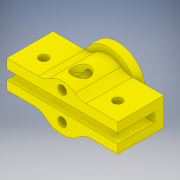
# Autodesk Inventor part: middledownthrustmt
Saved by Autodesk Inventor 2017 (Build 210142000, 142)
## iProperties
Created: 2017-08-12
Part Number: middledownthrustmt
Material: Generic
Document SubType Name: Modeling
Designer: Kai
Density: 1 g/cm^3
Appearance: Default
Author: Kai
Autodesk Inventor part; units mm, degrees
ref_plane "YZ Plane" through (0, 0, 0) normal (1, 0, 0) x (0, 1, 0)
ref_plane "XZ Plane" through (0, 0, 0) normal (0, 1, 0) x (-1, 0, 0)
ref_plane "XY Plane" through (0, 0, 0) normal (0, 0, 1) x (1, 0, 0)
sketch "Sketch1" plane through (0, 0, 0) normal (0, 0, 1) x (1, 0, 0)
  circle A0 centre (0, 0) radius 19.05
  dimension "d5" = 38.1
  constraints: 1 centre point
  measures "d5" diameter of A0
extrude "Extrusion1" add sketch "Sketch1" along normal blind 6.35
sketch "Sketch2" plane through (0, 0, 6.35) normal (0, 0, 1) x (1, 0, 0)
  line L0 (38.1, 9.525) -> (38.1, -9.525)
  line L1 (-38.1, -9.525) -> (-38.1, 9.525)
  line L2 (-34.9943, 0) -> (35.154, 0) construction
  line L3 (-38.1, 9.525) -> (-16.324, 9.525)
  line L4 (16.324, 9.525) -> (38.1, 9.525)
  line L5 (38.1, -9.525) -> (19.8184, -9.525)
  line L6 (-19.8184, -9.525) -> (-38.1, -9.525)
  arc A0 (-11.366, -12.7462) -> (11.366, -12.7462) centre (0, 0) ccw
  arc A1 (8.806, 11.9893) -> (-8.806, 11.9893) centre (0, 0) ccw
  arc A2 (-16.324, 9.525) -> (-8.806, 11.9893) centre (-16.324, 22.225) ccw
  arc A3 (8.806, 11.9893) -> (16.324, 9.525) centre (16.324, 22.225) ccw
  arc A4 (19.8184, -9.525) -> (11.366, -12.7462) centre (19.8184, -22.225) ccw
  arc A5 (-11.366, -12.7462) -> (-19.8184, -9.525) centre (-19.8184, -22.225) ccw
  point P0 (-11.4265, 9.525)
  point P1 (14.1749, -9.525)
  point P2 (-14.1749, -9.525)
  point P3 (11.4265, 9.525)
  dimension "d8" = 76.2
  dimension "d9" = 19.05
  dimension "d10" = 38.1
  dimension "d11" = 12.7
  dimension "d18" = 19.05
  constraints: 16 point on circle, 14 end point, 8 tangent, 6 centre point, 5 parallel, 4 point on line, 3 equal radius, 3 horizontal, 2 perpendicular, 1 coincident, 1 other
  measures "d8" distance of L0.end L1.start
  measures "d9" distance of L0.start L0.end
  measures "d10" distance from line of point (0, 0) L0
  measures "d11" radius of A2
  measures "d18" distance of L1.start L1.end
extrude "Extrusion2" add sketch "Sketch2" along normal blind 31.75
sketch "Sketch3" plane through (38.1, -9.525, 6.35) normal (1, 0, 0) x (0, 0, -1)
  line L0 (-31.75, 19.05) -> (-31.75, 0) projected
  line L1 (-31.75, 12.4336) -> (-6.35, 12.4336)
  line L2 (-6.35, 12.4336) -> (-6.35, 6.0836)
  line L3 (-6.35, 6.0836) -> (-31.75, 6.0836)
  line L4 (-31.75, 6.0836) -> (-31.75, 12.4336)
  line L5 (0, 19.05) -> (0, -0.5328) construction
  line L6 (0, 9.2586) -> (-14.0529, 9.2586) construction
  point P0 (6.35, 9.525)
  dimension "d14" = 25.4
  dimension "d15" = 6.35
  constraints: 10 end point, 3 parallel, 1 horizontal, 1 midpoint, 1 perpendicular, 1 point on line, 1 other
  measures "d14" distance of L2.end L3.end
  measures "d15" distance of L1.end L2.end
extrude "Extrusion3" cut sketch "Sketch3" against normal up to surface (76.2 mm away)
sketch "Sketch4" plane through (0, 0, 38.1) normal (0, 0, 1) x (1, 0, 0)
  circle A0 centre (0, 0) radius 9.5 construction
  circle A1 centre (0, 9.5) radius 1.6
  circle A2 centre (-9.5, 0) radius 1.6
  circle A3 centre (0, -9.5) radius 1.6
  circle A4 centre (9.5, 0) radius 1.6
  dimension "d19" = 19
  dimension "d20" = 3.2
  dimension "d23" = 360
  constraints: 4 centre point, 1 coincident, 1 vertical alignment, 11 other
  measures "d20" diameter of A1
extrude "Extrusion4" cut sketch "Sketch4" against normal up to surface (38.1 mm away)
sketch "Sketch5" plane through (0, 0, 38.1) normal (0, 0, 1) x (1, 0, 0)
  circle A0 centre (0, 9.5) radius 1.6 projected
  circle A1 centre (0, 9.5) radius 3
  circle A2 centre (-9.5, 0) radius 3
  circle A3 centre (0, -9.5) radius 3
  circle A4 centre (9.5, 0) radius 3
  point P0 (0, 0)
  dimension "d27" = 6
  dimension "d30" = 360
  constraints: 4 centre point, 1 coincident, 9 other
  measures "d27" diameter of A1
extrude "Extrusion5" cut sketch "Sketch5" against normal up to surface (31.75 mm away)
sketch "Sketch6" plane through (19.8184, -9.525, 6.35) normal (0, -1, 0) x (1, 0, 0)
  circle A0 centre (5.5816, 19.05) radius 3.1
  line L0 (18.2816, 0) -> (18.2816, 31.75) projected
  line L1 (0, 31.75) -> (18.2816, 31.75) projected
  line L2 (5.5816, 19.05) -> (-9.5835, 19.05) construction
  line L3 (-9.5835, 31.75) -> (-9.5835, 6.35) construction
  circle A1 centre (-19.8184, 19.05) radius 3.1
  circle A2 centre (-45.2184, 19.05) radius 3.1
  point P0 (-19.8184, -6.35)
  dimension "d34" = 6.2
  dimension "d35" = 12.7
  dimension "d36" = 12.7
  dimension "d39" = 25.4
  constraints: 3 centre point, 2 end point, 1 horizontal, 1 midpoint, 4 other
  measures "d34" diameter of A0
  measures "d35" distance from line of L0 L2.start
  measures "d36" distance from line of L2.start L1
  measures "d39" distance of L2.start A1.centre
extrude "Extrusion6" cut sketch "Sketch6" along normal mid plane 127
sketch "Sketch7" plane through (19.8184, -9.525, 6.35) normal (0, -1, 0) x (1, 0, 0)
  circle A0 centre (-19.8184, 19.05) radius 3.1 projected
  circle A1 centre (-19.8184, 19.05) radius 6
  point P0 (-19.8184, -6.35)
  dimension "d46" = 12
  constraints: 1 centre point, 1 coincident
  measures "d46" diameter of A1
extrude "Extrusion7" cut sketch "Sketch7" along normal blind 127
sketch "Sketch8" plane through (16.4978, 9.525, 6.35) normal (0, 1, 0) x (1, 0, 0)
  circle A0 centre (-16.4978, -19.05) radius 3.1 projected
  circle A1 centre (-16.4978, -19.05) radius 6
  point P0 (-16.4978, 6.35)
  dimension "d49" = 12
  constraints: 1 centre point, 1 coincident
  measures "d49" diameter of A1
extrude "Extrusion8" cut sketch "Sketch8" along normal blind 127 contours A0 | A1
body "Solid1"
